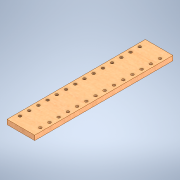
# Autodesk Inventor part: board
Saved by Autodesk Inventor 2022 (Build 260153000, 153)
## iProperties
Created: 2022-04-10
Part Number: board
Material: Wood (Cherry)
Document SubType Name: Modeling
Designer: Patrick
Density: 0.63 g/cm^3
Appearance: Cherry - Natural Low Gloss
Mass: 9.04921 g
Surface Area: 78.9376 cm^2
Volume: 14.3638 cm^3
Author: Patrick
Autodesk Inventor part; units mm, degrees
ref_plane "YZ Plane" through (0, 0, 0) normal (1, 0, 0) x (0, 1, 0)
ref_plane "XZ Plane" through (0, 0, 0) normal (0, 1, 0) x (-1, 0, 0)
ref_plane "XY Plane" through (0, 0, 0) normal (0, 0, 1) x (1, 0, 0)
sketch "Sketch1" plane through (0, 0, 0) normal (0, 1, 0) x (-1, 0, 0)
  line L0 (0, 0) -> (30, 0)
  line L1 (30, 0) -> (30, -150)
  line L2 (30, -150) -> (0, -150)
  line L3 (0, -150) -> (0, 0)
  dimension "d0" = 30
  dimension "d1" = 150
  constraints: 8 end point, 2 parallel, 1 horizontal, 1 perpendicular
  measures "d0" distance of L1.end L2.end
  measures "d1" distance of L0.end L1.end
extrude "Extrusion1" add sketch "Sketch1" along normal blind 5
sketch "Sketch2" plane through (0, 5, 0) normal (0, 1, 0) x (1, 0, 0)
  circle A0 centre (-26, 10) radius 1.5
  line L0 (-30, 0) -> (0, 0) projected
  line L1 (-30, 150) -> (-30, 0) projected
  circle A1 centre (-26, 20) radius 1.5
  circle A2 centre (-26, 30) radius 1.5
  circle A3 centre (-26, 40) radius 1.5
  circle A4 centre (-26, 50) radius 1.5
  circle A5 centre (-26, 60) radius 1.5
  circle A6 centre (-26, 70) radius 1.5
  circle A7 centre (-26, 80) radius 1.5
  circle A8 centre (-26, 90) radius 1.5
  circle A9 centre (-4, 10) radius 1.5
  circle A10 centre (-4, 20) radius 1.5
  circle A11 centre (-4, 30) radius 1.5
  circle A12 centre (-4, 40) radius 1.5
  circle A13 centre (-4, 50) radius 1.5
  circle A14 centre (-4, 60) radius 1.5
  circle A15 centre (-4, 70) radius 1.5
  circle A16 centre (-4, 80) radius 1.5
  circle A17 centre (-4, 90) radius 1.5
  circle A18 centre (-26, 100) radius 1.5
  circle A19 centre (-4, 100) radius 1.5
  circle A20 centre (-26, 110) radius 1.5
  circle A21 centre (-4, 110) radius 1.5
  circle A22 centre (-26, 120) radius 1.5
  circle A23 centre (-4, 120) radius 1.5
  circle A24 centre (-26, 130) radius 1.5
  circle A25 centre (-4, 130) radius 1.5
  circle A26 centre (-26, 140) radius 1.5
  circle A27 centre (-4, 140) radius 1.5
  dimension "d4" = 3
  dimension "d5" = 10
  dimension "d6" = 4
  dimension "d9" = 10
  dimension "d12" = 22
  constraints: 28 centre point, 1 horizontal, 1 vertical, 54 other
  measures "d4" diameter of A0
  measures "d5" distance from line of L0 A0.centre
  measures "d6" distance from line of L1 A0.centre
  measures "d9" distance of A0.centre A1.centre
  measures "d12" distance of A0.centre A9.centre
extrude "Extrusion2" cut sketch "Sketch2" against normal blind 5
body "Solid1"
